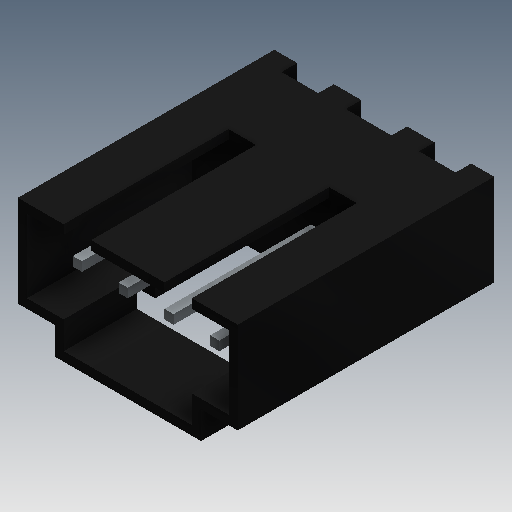
# Autodesk Inventor part: config - j9b1 connector
Saved by Autodesk Inventor 2019.1 (Build 231200000, 200)
## iProperties
Company: Autodesk Asia Pte. Ltd.
Created: 2005-12-05
Part Number: config - j9b1 connector
Document SubType Name: Modeling
Designer: Simon.Ng@autodesk.com
Stock Number: config - j9b1 connector
Density: 1 g/cm^3
Material: Generic
Mass: 0.404375 g
Surface Area: 8.9745 cm^2
Volume: 0.404375 cm^3
Appearance: Glossy - Black
Title: PC Demo
Author: Simon.Ng@autodesk.com
Autodesk Inventor part; units mm, degrees
ref_plane "YZ Plane" through (0, 0, 0) normal (1, 0, 0) x (0, 1, 0)
ref_plane "XZ Plane" through (0, 0, 0) normal (0, 1, 0) x (-1, 0, 0)
ref_plane "XY Plane" through (0, 0, 0) normal (0, 0, 1) x (1, 0, 0)
sketch "Sketch1" plane through (0, 0, 0) normal (0, 0, 1) x (1, 0, 0)
  line L0 (0, 6.95) -> (0, -2.15) construction
  line L1 (-7.2, 0) -> (9.6, 0) construction
  line L2 (-6, 0) -> (6, 0)
  line L3 (6, 0) -> (6, 5)
  line L4 (6, 5) -> (-6, 5)
  line L5 (-6, 5) -> (-6, 0)
  line L6 (-4, 0) -> (4, 0)
  line L7 (4, 0) -> (4, -1.5)
  line L8 (4, -1.5) -> (-4, -1.5)
  line L9 (-4, -1.5) -> (-4, 0)
  dimension "d0" = 12
  dimension "d1" = 5
  dimension "d2" = 1.5
  dimension "d3" = 8
  constraints: 16 end point, 4 parallel, 2 horizontal, 2 perpendicular, 2 point on line, 2 other
  measures "d0" distance of L3.end L4.end
  measures "d1" distance of L4.end L2.start
  measures "d2" distance of L8.end L6.start
  measures "d3" distance of L7.end L8.end
extrude "Extrusion1" add sketch "Sketch1" along normal blind 14
shell "Shell1" thickness 0.5 removed faces 1 at (-1.3333, 3.3333, 14) ; own thickness 5 on faces at (-1.3333, 3.3333, 0)
sketch "Sketch2" plane through (-4, -1.5, 0) normal (0, -1, 0) x (1, 0, 0)
  line L0 (8, 0) -> (8, 14) projected
  line L1 (0, 0) -> (8, 0)
  line L2 (8, 0) -> (8, 10)
  line L3 (8, 10) -> (0, 10)
  line L4 (0, 10) -> (0, 0)
  dimension "d7" = 10
  constraints: 8 end point, 2 parallel, 1 horizontal, 1 perpendicular, 1 point on line
  measures "d7" distance between parallel lines of L1 L3
extrude "Extrusion2" cut sketch "Sketch2" against normal up to surface (1.5 mm away)
sketch "Sketch3" plane through (4, -1.5, 10) normal (0, 0, -1) x (-1, 0, 0)
  line L0 (0.5, 1.5) -> (0.5, 2) projected
  line L1 (7.5, 2) -> (7.5, 1.5) projected
  line L2 (0.5, 2) -> (1.5, 2)
  line L3 (1.5, 2) -> (1.5, 1.5)
  line L4 (1.5, 1.5) -> (0.5, 1.5)
  line L5 (0.5, 1.5) -> (0.5, 2)
  line L6 (7.5, 2) -> (6.5, 2)
  line L7 (6.5, 2) -> (6.5, 1.5)
  line L8 (6.5, 1.5) -> (7.5, 1.5)
  line L9 (7.5, 1.5) -> (7.5, 2)
  line L10 (-2, 1.5) -> (10, 1.5) projected
  dimension "d11" = 1
  dimension "d12" = 1
  constraints: 16 end point, 4 parallel, 2 collinear, 2 horizontal, 2 perpendicular
  measures "d11" distance of L0.end L2.end
  measures "d12" distance of L1.start L6.end
extrude "Extrusion3" add sketch "Sketch3" along normal up to surface (5 mm away)
sketch "Sketch4" plane through (0, 0, 14) normal (0, 0, 1) x (1, 0, 0)
  line L0 (-5.5, 4.5) -> (5.5, 4.5) projected
  line L1 (-6, 5) -> (6, 5) projected
  line L2 (0, 6.95) -> (0, -2.15) projected
  line L3 (-3.5, 5) -> (-2, 5)
  line L4 (-2, 5) -> (-2, 4.5)
  line L5 (-2, 4.5) -> (-3.5, 4.5)
  line L6 (-3.5, 4.5) -> (-3.5, 5)
  line L7 (2, 5) -> (3.5, 5)
  line L8 (3.5, 5) -> (3.5, 4.5)
  line L9 (3.5, 4.5) -> (2, 4.5)
  line L10 (2, 4.5) -> (2, 5)
  dimension "d15" = 2
  dimension "d16" = 1.5
  constraints: 16 end point, 4 parallel, 4 point on line, 2 horizontal, 2 perpendicular, 2 other
  measures "d15" distance between parallel lines of L2 L4
  measures "d16" distance between parallel lines of L6 L4
extrude "Extrusion4" cut sketch "Sketch4" against normal up to surface (9 mm away) contours L6 L1 L4 L0 | L10 L1 L8 L0
sketch "Sketch5" plane through (-6, 5, 0) normal (0, 1, 0) x (1, 0, 0)
  line L0 (12, 0) -> (0, 0) projected
  line L1 (6, 1.4) -> (6, -18.2) projected
  line L2 (4.75, 0) -> (7.25, 0)
  line L3 (7.25, 0) -> (7.25, -0.85)
  line L4 (7.25, -0.85) -> (4.75, -0.85)
  line L5 (4.75, -0.85) -> (4.75, 0)
  line L6 (3.25, 0) -> (1.25, 0)
  line L7 (1.25, 0) -> (1.25, -0.85)
  line L8 (1.25, -0.85) -> (3.25, -0.85)
  line L9 (3.25, -0.85) -> (3.25, 0)
  line L10 (8.75, 0) -> (10.75, 0)
  line L11 (10.75, 0) -> (10.75, -0.85)
  line L12 (10.75, -0.85) -> (8.75, -0.85)
  line L13 (8.75, -0.85) -> (8.75, 0)
  dimension "d19" = 2.5
  dimension "d20" = 2
  dimension "d21" = 1.5
  dimension "d22" = 0.85
  constraints: 24 end point, 6 parallel, 3 horizontal, 3 perpendicular, 3 point on line, 2 collinear, 3 other
  measures "d19" distance of L3.end L4.end
  measures "d20" distance of L7.end L8.end
  measures "d21" distance between parallel lines of L5 L9
  measures "d22" distance of L6.end L7.end
extrude "Extrusion5" cut sketch "Sketch5" against normal through all
sketch "Sketch6" plane through (5.5, 0.5, 5) normal (0, 0, 1) x (1, 0, 0)
  line L0 (0, 0) -> (0, 4) construction
  line L1 (-11, 4) -> (-11, 0) construction
  line L2 (-5.5, 6.45) -> (-5.5, -2.65) construction
  line L3 (-11, 2) -> (0, 2) construction
  line L4 (-4.5, 2.25) -> (-4, 2.25)
  line L5 (-4, 2.25) -> (-4, 1.75)
  line L6 (-4, 1.75) -> (-4.5, 1.75)
  line L7 (-4.5, 1.75) -> (-4.5, 2.25)
  line L8 (-2, 2.25) -> (-1.5, 2.25)
  line L9 (-1.5, 2.25) -> (-1.5, 1.75)
  line L10 (-1.5, 1.75) -> (-2, 1.75)
  line L11 (-2, 1.75) -> (-2, 2.25)
  line L12 (-6.5, 2.25) -> (-7, 2.25)
  line L13 (-7, 2.25) -> (-7, 1.75)
  line L14 (-7, 1.75) -> (-6.5, 1.75)
  line L15 (-6.5, 1.75) -> (-6.5, 2.25)
  line L16 (-9, 2.25) -> (-9.5, 2.25)
  line L17 (-9.5, 2.25) -> (-9.5, 1.75)
  line L18 (-9.5, 1.75) -> (-9, 1.75)
  line L19 (-9, 1.75) -> (-9, 2.25)
  dimension "d25" = 1
  dimension "d26" = 0.5
  dimension "d27" = 2
  constraints: 34 end point, 8 parallel, 5 equal length, 4 horizontal, 4 perpendicular, 2 midpoint, 8 other
  measures "d25" distance between parallel lines of L2 L15
  measures "d26" distance of L12.start L12.end
  measures "d27" distance between parallel lines of L13 L19
extrude "Extrusion6" add sketch "Sketch6" along normal blind 8
equation "\"d12\" = d11"
body "Solid1"
